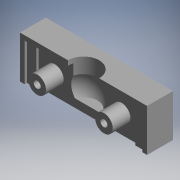
# Autodesk Inventor part: Part2v2
Saved by Autodesk Inventor 2017 (Build 210142000, 142)
## iProperties
Part Number: Part2v2
Material: Generic
Document SubType Name: Modeling
Designer: Ole Simmering
Appearance: Generic
Author: Ole Simmering
## iProperties of the stored document Part2v2_3DPrint.ipt
Part Number: Part2v2_3DPrint
Material: Generic
Document SubType Name: Modeling
Designer: Ole Simmering
Appearance: Generic
Author: Ole Simmering
Autodesk Inventor part; units mm, degrees
ref_plane "YZ Plane" through (0, 0, 0) normal (1, 0, 0) x (0, 1, 0)
ref_plane "XZ Plane" through (0, 0, 0) normal (0, 1, 0) x (-1, 0, 0)
ref_plane "XY Plane" through (0, 0, 0) normal (0, 0, 1) x (1, 0, 0)
sketch "Sketch1" plane through (0, 0, 0) normal (0, 0, 1) x (1, 0, 0)
  line L0 (0, 0) -> (27, 0)
  line L1 (27, 0) -> (27, 9)
  line L2 (27, 9) -> (0, 9)
  line L3 (0, 9) -> (0, 0)
  dimension "d0" = 27
  dimension "d1" = 9
  constraints: 8 end point, 2 parallel, 1 horizontal, 1 perpendicular
  measures "d0" distance of L2.end L1.end
  measures "d1" distance of L1.end L0.end
extrude "Extrusion1" add sketch "Sketch1" along normal blind 5
sketch "Sketch2" plane through (0, 0, 5) normal (0, 0, 1) x (1, 0, 0)
  line L0 (0, 0) -> (27, 0) projected
  line L1 (0, 0) -> (1, 0)
  line L2 (1, 0) -> (1, 8)
  line L3 (1, 8) -> (26, 8)
  line L4 (26, 8) -> (26, 0)
  line L5 (27, 0) -> (27, 9) projected
  line L6 (27, 0) -> (26, 0)
  line L7 (27, 0) -> (27, 9)
  line L8 (27, 9) -> (0, 9)
  line L9 (0, 9) -> (0, 0) projected
  line L10 (0, 9) -> (0, 0)
  line L11 (13.5, 12) -> (13.5, -6.262) construction
  dimension "d4" = 1
  dimension "d5" = 1
  constraints: 18 end point, 5 perpendicular, 2 point on line, 2 vertical, 1 collinear, 1 other
  measures "d4" distance of L0.start L1.end
  measures "d5" distance between parallel lines of L8 L3
extrude "Extrusion2" add sketch "Sketch2" along normal blind 0.5 contours L9 L8 L5 L0 L4 L3 L2
sketch "Sketch3" plane through (0, 0, 5) normal (0, 0, 1) x (1, 0, 0)
  line L0 (26, 0) -> (26, 8) construction
  line L1 (26, 8) -> (1, 8) construction
  line L2 (1, 8) -> (1, 0) construction
  line L3 (1, 0) -> (26, 0) construction
  line L4 (0, 0) -> (1, 0) construction
  line L5 (1, 0) -> (1, 8) construction
  line L6 (1, 8) -> (26, 8) construction
  line L7 (26, 8) -> (26, 0) construction
  line L8 (26, 0) -> (27, 0) construction
  line L9 (27, 0) -> (27, 9) construction
  line L10 (27, 9) -> (0, 9) construction
  line L11 (0, 9) -> (0, 0) construction
  line L12 (3, 0) -> (24, 0)
  line L13 (0, 0) -> (27, 0) projected
  line L14 (3, 0) -> (3, 8)
  line L15 (24, 0) -> (24, 8)
  line L16 (13.5, 10.7744) -> (13.5, -2.6721) construction
  line L17 (3, 8) -> (24, 8)
  dimension "d8" = 21
  constraints: 10 end point, 3 point on line, 1 horizontal, 1 parallel, 1 perpendicular, 1 vertical, 1 other
  measures "d8" distance of L12.start L12.end
extrude "Extrusion3" cut sketch "Sketch3" against normal blind 0.5
sketch "Sketch4" plane through (0, 0, 4.5) normal (0, 0, 1) x (1, 0, 0)
  line L0 (24, 0) -> (3, 0) construction
  line L1 (24, 8) -> (24, 0) construction
  line L2 (3, 8) -> (24, 8) construction
  line L3 (3, 0) -> (3, 8) construction
  line L4 (3, 0) -> (3, 8) construction
  line L5 (3, 8) -> (1, 8) construction
  line L6 (1, 8) -> (1, 0) construction
  line L7 (1, 0) -> (3, 0) construction
  line L8 (24, 8) -> (24, 0) construction
  line L9 (24, 0) -> (26, 0) construction
  line L10 (26, 0) -> (26, 8) construction
  line L11 (26, 8) -> (24, 8) construction
  line L12 (0, 0) -> (1, 0) construction
  line L13 (1, 0) -> (1, 8) construction
  line L14 (1, 8) -> (26, 8) construction
  line L15 (26, 8) -> (26, 0) construction
  line L16 (26, 0) -> (27, 0) construction
  line L17 (27, 0) -> (27, 9) construction
  line L18 (27, 9) -> (0, 9) construction
  line L19 (0, 9) -> (0, 0) construction
  line L20 (13.5, 12.5235) -> (13.5, -4.7396) construction
  circle A0 centre (6.4125, 4) radius 1.875
  circle A1 centre (20.5875, 4) radius 1.875
  point P0 (13.5, 10.4822)
  dimension "d12" = 4
  dimension "d13" = 14.175
  dimension "d14" = 3.75
  constraints: 2 centre point, 2 end point, 2 symmetric about line, 1 coincident, 1 point on line, 1 vertical, 2 other
  measures "d12" distance from line of L0 point (6.413, 4)
  measures "d13" diameter of point (6.413, 4) L20
  measures "d14" diameter of A0
extrude "Extrusion4" add sketch "Sketch4" along normal blind 3.75
sketch "Sketch5" plane through (6.4125, 4, 8.25) normal (0, 0, 1) x (1, 0, 0)
  circle A0 centre (0, 0) radius 1.875 projected
  circle A1 centre (14.175, 0) radius 1.875 projected
  point P0 (-6.4125, -4)
  constraints: 2 coincident
hole "Hole1" at (6.4125, 4, 8.25) at (20.5875, 4, 8.25) direction (0, 0, -1) diameter 1.5 depth 6 tip angle 118
sketch "Sketch7" plane through (0, 0, 5.5) normal (0, 0, 1) x (1, 0, 0)
  line L0 (0, 0) -> (1, 0) construction
  line L1 (1, 0) -> (1, 8) construction
  line L2 (1, 8) -> (26, 8) construction
  line L3 (26, 8) -> (26, 0) construction
  line L4 (26, 0) -> (27, 0) construction
  line L5 (27, 0) -> (27, 9) construction
  line L6 (27, 9) -> (0, 9) construction
  line L7 (0, 9) -> (0, 0) construction
  circle A0 centre (6.4125, 4) radius 1.875 construction
  circle A1 centre (20.5875, 4) radius 1.875 construction
  line L8 (24, 0) -> (3, 0) construction
  line L9 (24, 8) -> (24, 0) construction
  line L10 (3, 8) -> (24, 8) construction
  line L11 (3, 0) -> (3, 8) construction
  line L12 (24, 8) -> (24, 0) construction
  line L13 (24, 0) -> (26, 0) construction
  line L14 (26, 0) -> (26, 8) construction
  line L15 (26, 8) -> (24, 8) construction
  line L16 (3, 0) -> (3, 8) construction
  line L17 (3, 8) -> (1, 8) construction
  line L18 (1, 8) -> (1, 0) construction
  line L19 (1, 0) -> (3, 0) construction
  line L20 (27, 9) -> (0, 9) construction
  line L21 (13.5, 9) -> (13.5, 1.75)
  line L22 (23, 1.75) -> (16.5, 1.75) construction
  arc A2 (16.5, 1.75) -> (16.8166, 5.75) centre (13.5, 4) ccw
  line L23 (16.5, 1.75) -> (13.5, 1.75)
  line L24 (13.5, 1.75) -> (5.7709, 1.75) construction
  line L25 (16.8166, 5.75) -> (16.8166, 9)
  line L26 (16.8166, 9) -> (13.5, 9)
  line L27 (13.5, 1.75) -> (13.5, 0) construction
  dimension "d28" = 1.75
  dimension "d29" = 3.75
  dimension "d30" = 4
  dimension "d31" = 3
  constraints: 56 end point, 3 centre point, 3 horizontal, 2 midpoint, 2 point on circle, 2 point on line, 1 collinear, 1 perpendicular
  measures "d28" distance between parallel lines of L8 L22
  measures "d29" radius of A2
  measures "d30" vertical distance of L22.end L25.start
  measures "d31" distance of L22.end L21.end
revolve "Revolution1" cut sketch "Sketch7" angle 360 about axis through (13.5, 9, 5.5) along (0, -1, 0)
body "Solid1"
